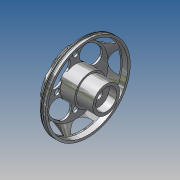
# Autodesk Inventor part: stator
Saved by Autodesk Inventor 2015 (Build 190159000, 159)
## iProperties
Created: 2016-12-08
Part Number: stator
Material: Allgemein
Document SubType Name: Modeling
Designer: NS
Density: 1 g/cm^3
Appearance: Default
RuleStatus: InUse
BeforeDocSave0: file://C:\_Vault_ausgecheckt\ilogic\ipt
Author: NS
Autodesk Inventor part; units mm, degrees
ref_plane "YZ Plane" through (0, 0, 0) normal (1, 0, 0) x (0, 1, 0)
ref_plane "XZ Plane" through (0, 0, 0) normal (0, 1, 0) x (-1, 0, 0)
ref_plane "XY Plane" through (0, 0, 0) normal (0, 0, 1) x (1, 0, 0)
sketch "Sketch1" plane through (0, 0, 0) normal (0, 1, 0) x (-1, 0, 0)
  line L0 (0, 0) -> (-30.3068, 0) construction
  line L1 (0, 0) -> (0, 26.4954) construction
  line L2 (0, 5.5) -> (-4, 5.5)
  line L3 (-4, 5.5) -> (-4, 2)
  line L4 (-4, 2) -> (-13, 2)
  line L5 (-13, 2) -> (-13, 5.5)
  line L6 (-13, 5.5) -> (-17, 5.5)
  line L7 (-17, 5.5) -> (-17, 7)
  line L8 (-17, 7) -> (-8.5, 7)
  line L9 (-8.5, 7) -> (-8.5, 8)
  line L10 (-8.5, 8) -> (-1, 8)
  line L11 (-1, 8) -> (-1, 17)
  line L12 (-1, 17) -> (-4.4, 20.9)
  line L13 (0, 5.5) -> (0, 18)
  line L14 (-7.4, 22.1) -> (-7.4, 20.9)
  line L15 (-7.4, 20.9) -> (-4.4, 20.9)
  line L16 (-6.2, 22.1) -> (-6.2, 21.4)
  line L17 (-6.2, 21.4) -> (-5.2, 21.4)
  line L18 (-5.2, 21.4) -> (-5.2, 22.1)
  line L19 (-4.5, 22.1) -> (-5.2, 22.1)
  line L20 (-6.2, 22.1) -> (-7.4, 22.1)
  arc A0 (-4.5, 22.1) -> (0, 17.6341) centre (10.403, 32.6166) ccw
  dimension "d2" = 2
  dimension "d3" = 4
  dimension "d4" = 4
  dimension "d5" = 17
  dimension "d6" = 4.5
  dimension "d7" = 5.5
  dimension "d8" = 1
  dimension "d9" = 20.9
  dimension "d11" = 3
  dimension "d12" = 1.2
  dimension "d13" = 2.9
  dimension "d14" = 18
  dimension "d15" = 4.5
  dimension "d16" = 9
  dimension "d17" = 7
  dimension "d18" = 8
  dimension "d19" = 0.7
  dimension "d20" = 1
  dimension "d21" = 0.7
  dimension "d22" = 18.24
  constraints: 42 end point, 13 perpendicular, 5 point on line, 2 horizontal, 2 point on circle, 1 centre point, 1 parallel, 1 vertical
  measures "d2" distance between parallel lines of L4 L0
  measures "d3" distance between parallel lines of L1 L3
  measures "d4" distance between parallel lines of L7 L5
  measures "d5" distance between parallel lines of L7 L1
  measures "d6" distance from line of L9.end L3
  measures "d7" distance between parallel lines of L0 L2
  measures "d8" distance between parallel lines of L1 L11
  measures "d9" distance from line of L0 L12.end
  measures "d11" distance of L14.end L12.end
  measures "d12" distance of L14.start L14.end
  measures "d13" distance of L19.start L14.start
  measures "d14" distance from line of L0 L13.end
  measures "d15" horizontal distance of L19.start L13.end
  measures "d16" distance from line of L10 L11.end
  measures "d17" distance between parallel lines of L0 L8
  measures "d18" distance between parallel lines of L0 L10
  measures "d19" distance from line of L18 L19.start
  measures "d20" distance of L16.end L17.end
  measures "d21" distance of L16.start L16.end
  measures "d22" radius of A0
revolve "Revolution1" add sketch "Sketch1" angle 360 about axis through (0, 0, 0) along (1, 0, 0)
fillet "Fillet1" radius 1 2 edges at (0, 0, -17.6341) (4.5, 0, -22.1)
sketch "Sketch2" plane through (0, 0, 0) normal (-1, 0, 0) x (0, 0, 1)
  circle A0 centre (0, 0) radius 22.1 projected
  line L0 (22.1, 0) -> (0, 0) construction
  line L1 (0, 0) -> (0, -22.1) construction
  arc A1 (5.9784, -10.4047) -> (9.9924, -6.6447) centre (0, 0) ccw construction
  arc A2 (7.9712, -13.873) -> (13.3232, -8.8596) centre (0, 0) ccw
  arc A3 (3.9856, -6.9365) -> (6.6616, -4.4298) centre (0, 0) ccw
  arc A4 (3.9856, -6.9365) -> (7.9712, -13.873) centre (5.9784, -10.4047) ccw
  arc A5 (13.3232, -8.8596) -> (6.6616, -4.4298) centre (9.9924, -6.6447) ccw
  line L2 (0, 0) -> (8.4853, -8.4853) construction
  line L3 (11.3137, -11.3137) -> (15.6271, -15.6271) construction
  arc A6 (13.873, 7.9712) -> (8.8596, 13.3232) centre (0, 0) ccw
  arc A7 (6.9365, 3.9856) -> (4.4298, 6.6616) centre (0, 0) ccw
  arc A8 (6.9365, 3.9856) -> (13.873, 7.9712) centre (10.4047, 5.9784) ccw
  arc A9 (8.8596, 13.3232) -> (4.4298, 6.6616) centre (6.6447, 9.9924) ccw
  arc A10 (-7.9712, 13.873) -> (-13.3232, 8.8596) centre (0, 0) ccw
  arc A11 (-3.9856, 6.9365) -> (-6.6616, 4.4298) centre (0, 0) ccw
  arc A12 (-3.9856, 6.9365) -> (-7.9712, 13.873) centre (-5.9784, 10.4047) ccw
  arc A13 (-13.3232, 8.8596) -> (-6.6616, 4.4298) centre (-9.9924, 6.6447) ccw
  arc A14 (-13.873, -7.9712) -> (-8.8596, -13.3232) centre (0, 0) ccw
  arc A15 (-6.9365, -3.9856) -> (-4.4298, -6.6616) centre (0, 0) ccw
  arc A16 (-6.9365, -3.9856) -> (-13.873, -7.9712) centre (-10.4047, -5.9784) ccw
  arc A17 (-8.8596, -13.3232) -> (-4.4298, -6.6616) centre (-6.6447, -9.9924) ccw
  arc A18 (19.5213, -10.3599) -> (9.4052, -19.9988) centre (17.1518, -18.001) ccw
  arc A19 (21.1292, 6.4781) -> (20.7918, -7.4908) centre (24.8567, -0.6005) ccw
  arc A20 (10.3599, 19.5213) -> (19.9988, 9.4052) centre (18.001, 17.1518) ccw
  arc A21 (-6.4781, 21.1292) -> (7.4908, 20.7918) centre (0.6005, 24.8567) ccw
  arc A22 (-19.5213, 10.3599) -> (-9.4052, 19.9988) centre (-17.1518, 18.001) ccw
  arc A23 (-21.1292, -6.4781) -> (-20.7918, 7.4908) centre (-24.8567, 0.6005) ccw
  arc A24 (-10.3599, -19.5213) -> (-19.9988, -9.4052) centre (-18.001, -17.1518) ccw
  arc A25 (6.4781, -21.1292) -> (-7.4908, -20.7918) centre (-0.6005, -24.8567) ccw
  arc A26 (20.7918, -7.4908) -> (21.1292, 6.4781) centre (0, 0) ccw
  arc A27 (9.4052, -19.9988) -> (19.5213, -10.3599) centre (0, 0) ccw
  arc A28 (-7.4908, -20.7918) -> (6.4781, -21.1292) centre (0, 0) ccw
  arc A29 (-19.9988, -9.4052) -> (-10.3599, -19.5213) centre (0, 0) ccw
  arc A30 (-20.7918, 7.4908) -> (-21.1292, -6.4781) centre (0, 0) ccw
  arc A31 (-9.4052, 19.9988) -> (-19.5213, 10.3599) centre (0, 0) ccw
  arc A32 (19.9988, 9.4052) -> (10.3599, 19.5213) centre (0, 0) ccw
  arc A33 (7.4908, 20.7918) -> (-6.4781, 21.1292) centre (0, 0) ccw
  point P0 (0, 0)
  point P1 (11.3137, 11.3137)
  point P2 (-11.3137, 11.3137)
  point P3 (-11.3137, -11.3137)
  dimension "d26" = 5.5
  dimension "d27" = 16
  dimension "d28" = 8
  dimension "d31" = 360
  dimension "d35" = 8
  dimension "d38" = 360
  constraints: 77 point on circle, 33 centre point, 8 end point, 4 tangent, 2 coincident, 1 horizontal, 1 perpendicular, 82 other
  measures "d26" distance of A1.start A1.end
  measures "d27" radius of A2
  measures "d28" radius of A3
  measures "d35" radius of A18
extrude "Extrusion1" cut sketch "Sketch2" against normal blind 4 contours A0 A19 | A20 A0 | A0 A18 | A21 A0 | A0 A25 | A22 A0 | A0 A24 | A23 A0 | A4 A3 A5 A2 | A8 A7 A9 A6 | A12 A11 A13 A10 | A16 A15 A17 A14
sketch "Sketch3" plane through (0, 0, 0) normal (-1, 0, 0) x (0, -0.4048834, 0.9143683)
  circle A0 centre (0, 0) radius 2 projected
  circle A1 centre (0, 0) radius 12.5 construction
  circle A2 centre (0, 0) radius 9.5 construction
  line L0 (0, 0) -> (17.6881, 7.858) construction
  line L1 (0, 0) -> (-19.3723, 43.6064) construction
  circle A3 centre (11.4235, 5.0749) radius 1.5
  circle A4 centre (-3.8569, 8.6818) radius 1.5
  circle A5 centre (-11.4235, -5.0749) radius 1.5
  circle A6 centre (3.8569, -8.6818) radius 1.5
  point P0 (0, 0)
  dimension "d42" = 25
  dimension "d43" = 19
  dimension "d44" = 3
  dimension "d45" = 3
  constraints: 4 centre point, 4 end point, 2 coincident, 2 point on line, 2 symmetric about line, 8 other
  measures "d44" diameter of A3
  measures "d45" diameter of A4
extrude "Extrusion2" cut sketch "Sketch3" against normal through all contours A3 | A4 | A5 | A6
body "Solid1"
